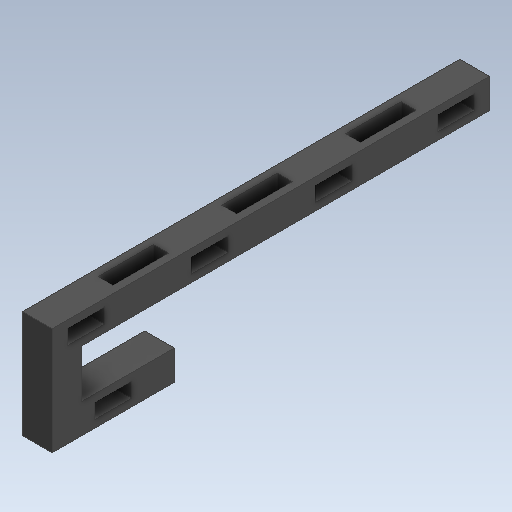
# Autodesk Inventor part: spool holder
Saved by Autodesk Inventor 2020.2 (Build 242310000, 310)
## iProperties
Created: 2020-02-05
Part Number: spool holder
Material: PLA
Document SubType Name: Modeling
Designer: mulve
Density: 1.3 g/cm^3
Appearance: Generic
Mass: 19.875 g
Surface Area: 107.288 cm^2
Volume: 15.2885 cm^3
Author: mulve
Autodesk Inventor part; units mm, degrees
ref_plane "YZ Plane" through (0, 0, 0) normal (1, 0, 0) x (0, 1, 0)
ref_plane "XZ Plane" through (0, 0, 0) normal (0, 1, 0) x (-1, 0, 0)
ref_plane "XY Plane" through (0, 0, 0) normal (0, 0, 1) x (1, 0, 0)
sketch "Sketch1" plane through (0, 0, 0) normal (1, 0, 0) x (0, 1, 0)
  line L0 (0, 0) -> (0, -139.8524)
  line L1 (0, 0) -> (-16.51, 0)
  line L2 (-16.51, 0) -> (-16.51, -31.75)
  line L3 (-16.51, -31.75) -> (-26.67, -31.75)
  line L4 (-26.67, -31.75) -> (-26.67, 10.16)
  line L5 (-26.67, 10.16) -> (10.16, 10.16)
  line L6 (10.16, 10.16) -> (10.16, -139.8524)
  line L7 (10.16, -139.8524) -> (0, -139.8524)
  dimension "d1" = 10.16
  dimension "d2" = 10.16
  dimension "d3" = 16.51
  dimension "d4" = 31.75
  dimension "d5" = 10.16
  dimension "d17" = 150.0124
  constraints: 16 end point, 6 perpendicular, 1 horizontal, 1 parallel, 1 vertical
  measures "d1" distance of L6.end L0.end
  measures "d2" distance between parallel lines of L5 L1
  measures "d3" distance of L0.start L1.end
  measures "d4" distance of L1.end L2.end
  measures "d5" distance of L2.end L3.end
  measures "d17" distance between parallel lines of L7 L5
extrude "Extrusion1" add sketch "Sketch1" along normal blind 10.16
sketch "Sketch2" plane through (0, 10.16, 10.16) normal (0, 1, 0) x (1, 0, 0)
  line L0 (2.54, 23.3934) -> (7.62, 23.3934)
  line L1 (7.62, 23.3934) -> (7.62, 42.4434)
  line L2 (7.62, 42.4434) -> (2.54, 42.4434)
  line L3 (2.54, 42.4434) -> (2.54, 23.3934)
  line L4 (0, 0) -> (10.16, 0) projected
  line L5 (0, 150.0124) -> (0, 0) projected
  line L6 (10.16, 150.0124) -> (10.16, 0) projected
  line L7 (2.54, 65.8368) -> (7.62, 65.8368)
  line L8 (7.62, 65.8368) -> (7.62, 84.8868)
  line L9 (7.62, 84.8868) -> (2.54, 84.8868)
  line L10 (2.54, 84.8868) -> (2.54, 65.8368)
  line L11 (2.54, 108.2802) -> (7.62, 108.2802)
  line L12 (7.62, 108.2802) -> (7.62, 127.3302)
  line L13 (7.62, 127.3302) -> (2.54, 127.3302)
  line L14 (2.54, 127.3302) -> (2.54, 108.2802)
  line L15 (0, 150.0124) -> (10.16, 150.0124) projected
  point P0 (0, 10.16)
  dimension "d8" = 23.3934
  dimension "d9" = 19.05
  dimension "d10" = 5.08
  dimension "d11" = 2.54
  dimension "d12" = 2.54
  dimension "d13" = 19.05
  dimension "d14" = 23.3934
  dimension "d15" = 19.05
  dimension "d16" = 23.3934
  dimension "d18" = 22.6822
  dimension "d19" = 5.08
  dimension "d20" = 5.08
  dimension "d21" = 2.54
  dimension "d22" = 2.54
  dimension "d23" = 2.54
  dimension "d24" = 2.54
  constraints: 24 end point, 6 parallel, 3 horizontal, 3 perpendicular
  measures "d8" distance between parallel lines of L4 L0
  measures "d9" distance of L2.end L0.start
  measures "d10" distance of L1.end L2.end
  measures "d11" distance between parallel lines of L5 L3
  measures "d12" distance between parallel lines of L6 L1
  measures "d13" distance of L9.end L7.start
  measures "d14" distance between parallel lines of L7 L2
  measures "d15" distance of L13.end L11.start
  measures "d16" distance between parallel lines of L11 L9
  measures "d18" distance between parallel lines of L15 L13
  measures "d19" distance of L8.end L9.end
  measures "d20" distance of L11.start L11.end
  measures "d21" distance between parallel lines of L5 L14
  measures "d22" distance between parallel lines of L6 L12
  measures "d23" distance between parallel lines of L5 L10
  measures "d24" distance between parallel lines of L6 L8
extrude "Extrusion2" cut sketch "Sketch2" against normal blind 10.16 contours L3 L2 L1 L0 | L10 L9 L8 L7 | L14 L13 L12 L11
sketch "Sketch3" plane through (10.16, 0, 0) normal (1, 0, 0) x (0, 0, -1)
  line L0 (17.145, -24.13) -> (4.445, -24.13)
  line L1 (4.445, -24.13) -> (4.445, -19.05)
  line L2 (4.445, -19.05) -> (17.145, -19.05)
  line L3 (17.145, -19.05) -> (17.145, -24.13)
  line L4 (31.75, -16.51) -> (0, -16.51) projected
  line L5 (-10.16, -26.67) -> (31.75, -26.67) projected
  line L6 (-10.16, 10.16) -> (-10.16, -26.67) projected
  line L7 (31.75, -26.67) -> (31.75, -16.51) projected
  line L8 (-4.8133, 7.62) -> (7.8867, 7.62)
  line L9 (7.8867, 7.62) -> (7.8867, 2.54)
  line L10 (7.8867, 2.54) -> (-4.8133, 2.54)
  line L11 (-4.8133, 2.54) -> (-4.8133, 7.62)
  line L12 (139.8524, 10.16) -> (-10.16, 10.16) projected
  line L13 (0, 0) -> (139.8524, 0) projected
  line L14 (134.8613, 2.54) -> (122.1613, 2.54)
  line L15 (122.1613, 2.54) -> (122.1613, 7.62)
  line L16 (122.1613, 7.62) -> (134.8613, 7.62)
  line L17 (134.8613, 7.62) -> (134.8613, 2.54)
  line L18 (139.8524, 0) -> (139.8524, 10.16) projected
  line L19 (80.0735, 7.62) -> (92.7735, 7.62)
  line L20 (92.7735, 7.62) -> (92.7735, 2.54)
  line L21 (92.7735, 2.54) -> (80.0735, 2.54)
  line L22 (80.0735, 2.54) -> (80.0735, 7.62)
  line L23 (37.6301, 7.62) -> (50.3301, 7.62)
  line L24 (50.3301, 7.62) -> (50.3301, 2.54)
  line L25 (50.3301, 2.54) -> (37.6301, 2.54)
  line L26 (37.6301, 2.54) -> (37.6301, 7.62)
  point P0 (13.2334, 10.16)
  point P1 (117.1702, 10.16)
  point P2 (55.6768, 10.16)
  point P3 (32.2834, 10.16)
  point P4 (74.7268, 10.16)
  point P5 (98.1202, 10.16)
  dimension "d27" = 12.7
  dimension "d28" = 2.54
  dimension "d29" = 5.08
  dimension "d30" = 2.54
  dimension "d31" = 14.605
  dimension "d32" = 14.605
  dimension "d33" = 5.3467
  dimension "d34" = 12.7
  dimension "d35" = 5.3467
  dimension "d36" = 5.08
  dimension "d37" = 2.54
  dimension "d38" = 2.54
  dimension "d39" = 5.08
  dimension "d40" = 4.9911
  dimension "d41" = 12.7
  dimension "d42" = 4.9911
  dimension "d43" = 2.54
  dimension "d44" = 2.54
  dimension "d45" = 12.7
  dimension "d46" = 5.3467
  dimension "d47" = 5.3467
  dimension "d48" = 12.7
  dimension "d49" = 5.3467
  dimension "d50" = 5.3467
  constraints: 40 end point, 10 parallel, 5 horizontal, 5 perpendicular, 2 point on line
  measures "d27" distance of L1.end L2.end
  measures "d28" distance between parallel lines of L4 L2
  measures "d29" distance of L2.end L0.start
  measures "d30" distance between parallel lines of L5 L0
  measures "d31" distance between parallel lines of L6 L1
  measures "d32" distance between parallel lines of L7 L3
  measures "d33" distance from line of point (13.233, 10.16) L9
  measures "d34" distance of L8.start L8.end
  measures "d35" distance between parallel lines of L6 L11
  measures "d36" distance of L10.end L8.start
  measures "d37" distance between parallel lines of L12 L8
  measures "d38" distance between parallel lines of L13 L10
  measures "d39" distance of L16.end L14.start
  measures "d40" distance from line of L15 point (117.17, 10.16)
  measures "d41" distance of L15.end L16.end
  measures "d42" distance between parallel lines of L18 L17
  measures "d43" distance between parallel lines of L12 L16
  measures "d44" distance between parallel lines of L13 L14
  measures "d45" distance of L23.start L23.end
  measures "d46" distance from line of point (55.677, 10.16) L24
  measures "d47" distance from line of L26 point (32.283, 10.16)
  measures "d48" distance of L19.start L19.end
  measures "d49" distance from line of point (74.727, 10.16) L22
  measures "d50" distance from line of L20 point (98.12, 10.16)
extrude "Extrusion3" cut sketch "Sketch3" against normal through all
equation "\"d2\" = d1"
equation "\"d11\" = d12"
equation "\"d13\" = d9"
equation "\"d14\" = d8"
equation "\"d15\" = d13"
equation "\"d16\" = d14"
equation "\"d28\" = d30"
equation "\"d31\" = d32"
equation "\"d33\" = d35"
equation "\"d37\" = d38"
equation "\"d40\" = d42"
equation "\"d43\" = d44"
equation "\"d46\" = d47"
equation "\"d49\" = d50"
body "Solid1"
